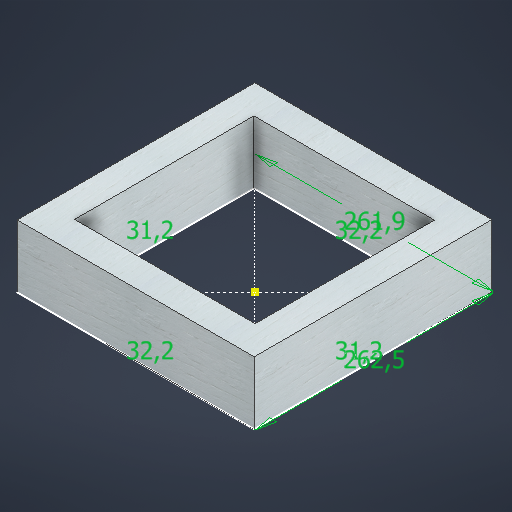
# Autodesk Inventor part: NinhoColmeia
Saved by Autodesk Inventor 2027 (Build 310192000, 192)
## iProperties
Created: 2026-10-01
Part Number: NinhoColmeia
Material: Genérico
Document SubType Name: Modeling
Designer: EspacoMaker
Density: 1 g/cm^3
Appearance: Padrão
Author: EspacoMaker
Autodesk Inventor part; units mm, degrees
ref_plane "YZ Plane" through (0, 0, 0) normal (1, 0, 0) x (0, 1, 0)
ref_plane "XZ Plane" through (0, 0, 0) normal (0, 1, 0) x (-1, 0, 0)
ref_plane "XY Plane" through (0, 0, 0) normal (0, 0, 1) x (1, 0, 0)
sketch "Esboço1" plane through (0, 0, 0) normal (0, 1, 0) x (-1, 0, 0)
  line L0 (130.95, 131.25) -> (-130.95, 131.25)
  line L1 (-130.95, 131.25) -> (-130.95, -131.25)
  line L2 (-130.95, -131.25) -> (130.95, -131.25)
  line L3 (130.95, -131.25) -> (130.95, 131.25)
  line L4 (130.95, 131.25) -> (-130.95, -131.25) construction
  line L5 (-130.95, 131.25) -> (130.95, -131.25) construction
  line L6 (130.95, 99.05) -> (-130.95, 99.05)
  line L7 (-130.95, -99.05) -> (130.95, -99.05)
  line L8 (-99.75, 131.25) -> (-99.75, -131.25)
  line L9 (99.75, -131.25) -> (99.75, 131.25)
  point P0 (0, 0)
  point P1 (99.75, -99.05)
  point P2 (99.75, 99.05)
  point P3 (-99.75, 99.05)
  point P4 (-99.75, -99.05)
  dimension "d0" = 261.9
  dimension "d1" = 262.5
  dimension "d2" = 32.2
  dimension "d3" = 32.2
  dimension "d4" = 31.2
  dimension "d5" = 31.2
  constraints: 20 end point, 6 parallel, 2 midpoint, 1 horizontal, 1 perpendicular
  measures "d0" distance of L2.end L1.end
  measures "d1" distance of L1.end L0.end
  measures "d2" distance between parallel lines of L0 L6
  measures "d3" distance between parallel lines of L2 L7
  measures "d4" distance between parallel lines of L1 L8
  measures "d5" distance between parallel lines of L3 L9
extrude "Extrusão1" add sketch "Esboço1" along normal blind 69.3
extrude "Extrusão2" cut sketch "Esboço1" along normal blind 69.3 contours L9 L7 L8 L6
